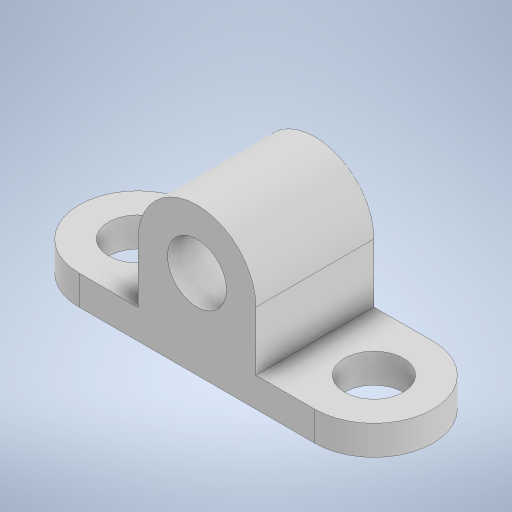
# Autodesk Inventor part: LAB1LLCT
Saved by Autodesk Inventor 2024 (Build 280153000, 153)
## iProperties
Created: 2024-02-04
Part Number: LAB1LLCT
Material: Generic
Document SubType Name: Sheet Metal
Designer: Admin
Density: 1 g/cm^3
Sheet Metal Rule: Default
Appearance: Default
Author: Admin
Autodesk Inventor part; units mm, degrees
ref_plane "YZ Plane" through (0, 0, 0) normal (1, 0, 0) x (0, 1, 0)
ref_plane "XZ Plane" through (0, 0, 0) normal (0, 1, 0) x (-1, 0, 0)
ref_plane "XY Plane" through (0, 0, 0) normal (0, 0, 1) x (1, 0, 0)
sketch "Sketch1" plane through (0, 0, 0) normal (0, 0, 1) x (1, 0, 0)
  line L0 (1016, 0) -> (-1016, 0)
  line L1 (-1016, 0) -> (-1016, 254)
  line L2 (-1016, 0) -> (-762, 0) construction
  line L3 (-1016, 254) -> (-508, 254)
  line L4 (-508, 254) -> (-508, 762)
  line L5 (1016, 0) -> (1016, 254)
  line L6 (1016, 254) -> (508, 254)
  line L7 (508, 254) -> (508, 762)
  arc A0 (508, 762) -> (-508, 762) centre (0, 762) ccw
  circle A1 centre (0, 762) radius 254
  point P0 (0, 0)
  dimension "d7" = 2032
  dimension "d8" = 254
  dimension "d10" = 508
  dimension "d12" = 508
  dimension "d19" = 254
  dimension "d20" = 508
  dimension "d21" = 508
  dimension "d22" = 508
  constraints: 16 end point, 5 perpendicular, 2 centre point, 2 horizontal, 2 point on circle, 2 vertical, 1 coincident
  measures "d7" distance of L0.start L0.end
  measures "d8" distance of L0.end L1.end
  measures "d10" distance of L1.end L3.end
  measures "d12" distance of L3.end L4.end
  measures "d19" distance of L0.start L5.end
  measures "d20" distance of L5.end L6.end
  measures "d21" distance of L6.end L7.end
  measures "d22" diameter of A1
extrude "Extrusion1" add sketch "Sketch1" against normal blind 1016 contours L0 L1 L3 L4 A0 L7 L6 L5 | A1
sketch "Sketch2" plane through (0, 0, 0) normal (0, 0, 1) x (1, 0, 0)
  arc A0 (508, 762) -> (-508, 762) centre (0, 762) ccw projected
  circle A1 centre (0, 762) radius 254
  point P0 (0, 0)
  dimension "d25" = 508
  constraints: 1 centre point, 1 coincident
  measures "d25" diameter of A1
extrude "Extrusion2" cut sketch "Sketch2" against normal blind 1016
sketch "Sketch3" plane through (508, 254, 0) normal (0, 1, 0) x (1, 0, 0)
  line L0 (-1524, 0) -> (-1524, 1016) projected
  arc A0 (-1524, 1016) -> (-1524, 0) centre (-1524, 508) ccw
  line L1 (508, 0) -> (508, 1016) projected
  arc A1 (508, 0) -> (508, 1016) centre (508, 508) ccw
  circle A2 centre (-1524, 508) radius 254
  circle A3 centre (508, 508) radius 254
  point P0 (-508, 0)
  point P1 (508, 762)
  point P2 (508, 254)
  point P3 (-1524, 254)
  point P4 (-1524, 762)
  dimension "d28" = 508
  dimension "d29" = 508
  constraints: 4 centre point, 4 point on circle, 2 coincident, 2 midpoint
  measures "d28" diameter of A2
  measures "d29" diameter of A3
extrude "Extrusion3" add sketch "Sketch3" against normal blind 254 contours A0 L0 A2 | L1 A3 A1
sketch "Sketch4" plane through (-508, 254, 0) normal (0, 1, 0) x (1, 0, 0)
  line L0 (-508, 254) -> (-508, 762) projected
  circle A0 centre (-508, 508) radius 254
  line L1 (1524, 254) -> (1524, 762) projected
  arc A1 (1524, 254) -> (1524, 762) centre (1524, 508) ccw projected
  circle A2 centre (1524, 508) radius 254
  point P0 (508, 0)
  constraints: 2 midpoint, 6 other
extrude "Extrusion4" cut sketch "Sketch4" against normal blind 254 contours L0 A0 | A2 L1 picked at (-364.7512, 468.4995)
equation "\"BendRadius\" = Thickness"
equation "\"BendReliefWidth\" = Thickness"
equation "\"BendReliefDepth\" = 0.5 * Thickness"
equation "\"CornerReliefSize\" = 4 * Thickness"
equation "\"MinimumRemnant\" = 2 * Thickness"
equation "\"TransitionRadius\" = BendRadius"
equation "\"JacobiRadiusSize\" = BendRadius"
equation "\"GapSize\" = Thickness"
equation "\"Thickness\" = 3.048"
body "Solid1"
